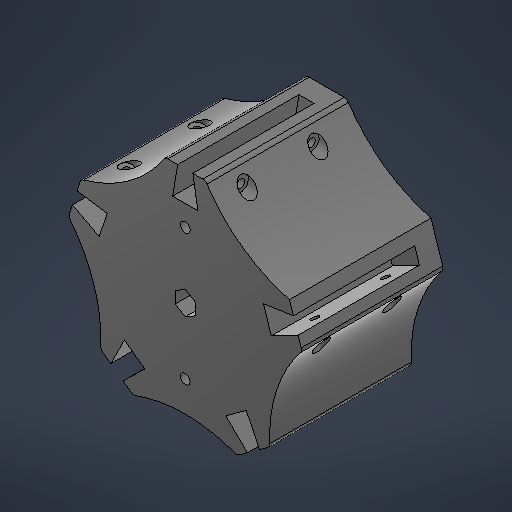
# Autodesk Inventor part: 3DPRINT,HUB
Saved by Autodesk Inventor 2026.1 (Build 301233020, 233B)
## iProperties
Created: 2026-02-05
Part Number: 3DPRINT,HUB
Material: ABS Plastic
Document SubType Name: Modeling
Designer: Owen L
Density: 0.316929 g/cm^3
Appearance: Smooth - Black
Mass: 362.874 g
Surface Area: 937.42 cm^2
Volume: 1144.97 cm^3
Author: Owen L
Autodesk Inventor part; units mm, degrees
ref_plane "XZ Plane" through (0, 0, 0) normal (0, 1, 0) x (-1, 0, 0)
ref_plane "XY Plane" through (0, 0, 0) normal (0, 0, 1) x (1, 0, 0)
sketch "Sketch1" plane through (0, 0, 0) normal (0, 0, 1) x (1, 0, 0)
  line L0 (0, 0) -> (0, 73.025) construction
  line L1 (-12.7, 73.025) -> (12.7, 73.025)
  line L2 (-73.3754, 10.4875) -> (-65.5264, 34.6444)
  line L3 (-32.6485, -66.5433) -> (-53.1975, -51.6136)
  line L4 (53.1975, -51.6136) -> (32.6485, -66.5433)
  line L5 (65.5264, 34.6444) -> (73.3754, 10.4875)
  arc A0 (12.7, 73.025) -> (65.5264, 34.6444) centre (87.7159, 120.7306) ccw
  arc A1 (73.3754, 10.4875) -> (53.1975, -51.6136) centre (141.9273, -46.115) ccw
  arc A2 (32.6485, -66.5433) -> (-32.6485, -66.5433) centre (0, -149.2312) ccw
  arc A3 (-53.1975, -51.6136) -> (-73.3754, 10.4875) centre (-141.9273, -46.115) ccw
  arc A4 (-65.5264, 34.6444) -> (-12.7, 73.025) centre (-87.7159, 120.7306) ccw
  point P0 (65.5264, 34.6444)
  dimension "d0" = 73.025
  dimension "d1" = 25.4
  dimension "d4" = 360
  dimension "d6" = 88.9
  constraints: 12 end point, 10 point on circle, 5 centre point, 4 equal radius, 1 coincident, 1 horizontal, 1 midpoint, 1 vertical, 16 other
  measures "d0" distance of L0.start L0.end
  measures "d1" distance of L1.start L1.end
  measures "d6" radius of A0
extrude "Extrusion5" add sketch "Sketch1" along normal mid plane 88.9
ref_plane "Work Plane5" through (0, 0, 44.45) normal (0, 0, 1) x (1, 0, 0)
sketch "Sketch7" plane through (0, 0, 44.45) normal (0, 0, 1) x (1, 0, 0)
  line L0 (12.7, 73.025) -> (-12.7, 73.025) projected
  line L1 (0, 0) -> (0, 73.025) construction
  line L2 (-4.7625, 73.025) -> (-7.9375, 54.2414)
  line L3 (-7.9375, 54.2414) -> (7.9375, 54.2414)
  line L4 (7.9375, 54.2414) -> (4.7625, 73.025)
  dimension "d121" = 19.05
  dimension "d122" = 15.875
  dimension "d147" = 9.525
  constraints: 8 end point, 2 point on line, 1 equal length, 1 midpoint, 1 other
  measures "d121" distance of L2.start L2.end
  measures "d122" distance of L2.end L3.end
  measures "d147" distance of L2.start L4.end
extrude "Extrusion6" cut sketch "Sketch7" against normal blind 76.2
pattern_circular "Circular Pattern3" count 5 over 360 about axis through (0, 0, -10) along (0, 0, 1) of "Extrusion6"
fillet "Fillet3" radius 3.175 9 edges at (-73.3754, 10.4875, 0) (-65.5264, 34.6444, 0) (-12.7, 73.025, 0) (-53.1975, -51.6136, 0) (-32.6485, -66.5433, 0) (32.6485, -66.5433, 0) (53.1975, -51.6136, 0) (73.3754, 10.4875, 0) (12.7, 73.025, 0)
sketch "Sketch9" plane through (0, 0, -44.45) normal (0, 0, -1) x (-1, 0, 0)
  point P0 (0, 0)
  point P1 (0, -44.45)
  point P2 (38.4948, -22.225)
  point P3 (38.4948, 22.225)
  point P4 (0, 44.45)
  point P5 (-38.4948, 22.225)
  point P6 (-38.4948, -22.225)
  dimension "d93" = 44.45
  dimension "d96" = 360
  constraints: 1 vertical alignment, 7 other
  measures "d93" distance of point (0, 0) point (0, -44.45)
hole "Hole1" at (0, -44.45, -44.45) at (-38.4948, -22.225, -44.45) at (-38.4948, 22.225, -44.45) at (0, 44.45, -44.45) at (38.4948, 22.225, -44.45) at (38.4948, -22.225, -44.45) direction (0, 0, 1) diameter 6.12 depth 12.7 tip angle 118
sketch "Sketch10" plane through (0, 0, 44.45) normal (0, 0, 1) x (1, 0, 0)
  line L0 (0, 41.275) -> (0, 0) construction
  point P0 (0, -41.275)
  dimension "d107" = 360
  dimension "d109" = 41.275
  constraints: 2 end point, 1 vertical, 3 other
  measures "d109" distance of L0.start L0.end
hole "Hole2" at (0, 41.275, 44.45) at (0, -41.275, 44.45) direction (0, 0, -1) diameter 6.12 depth 12.7 tip angle 118
sketch "Sketch11" plane through (0, 0, -44.45) normal (0, 0, -1) x (-1, 0, 0)
  line L0 (-6.4135, -3.7028) -> (-6.4135, 3.7028)
  line L1 (-6.4135, 3.7028) -> (0, 7.4057)
  line L2 (0, 7.4057) -> (6.4135, 3.7028)
  line L3 (6.4135, 3.7028) -> (6.4135, -3.7028)
  line L4 (6.4135, -3.7028) -> (0, -7.4057)
  line L5 (0, -7.4057) -> (-6.4135, -3.7028)
  point P0 (0, 0)
  point P1 (0, 0)
  dimension "d118" = 12.827
  constraints: 12 end point, 1 coincident, 1 vertical, 13 other
  measures "d118" distance between parallel lines of L3 L0
extrude "Extrusion8" cut sketch "Sketch11" against normal through all
ref_plane "Work Plane6" through (38.1, 0, 0) normal (1, 0, 0) x (0, 1, 0)
sketch "Sketch12" plane through (38.1, 0, 0) normal (1, 0, 0) x (0, 1, 0)
  line L0 (71.6045, -44.45) -> (35.0827, -44.45) projected
  circle A0 centre (63.5, 25.4) radius 2.5527
  circle A1 centre (63.5, -19.05) radius 2.5527
  point P0 (0, 0)
  dimension "d123" = 63.5
  dimension "d124" = 25.4
  dimension "d125" = 44.45
  dimension "d127" = 5.1054
  constraints: 2 centre point, 2 coincident, 1 equal radius, 1 vertical alignment
  measures "d123" horizontal distance of point (0, 0) point (63.5, -19.05)
  measures "d124" distance from line of L0 point (63.5, -19.05)
  measures "d125" distance of point (63.5, -19.05) point (63.5, 25.4)
  measures "d127" diameter of A0
hole "Hole3" at (38.1, 63.5, 25.4) at (38.1, 63.5, -19.05) direction (-1, 0, 0) diameter 4.9784 depth 34.925 tip angle 118 counterbore diameter 9.779 counterbore depth 22.352
ref_plane "Work Plane7" through (-38.1, 0, 0) normal (1, 0, 0) x (0, 1, 0)
sketch "Sketch13" plane through (-38.1, 0, 0) normal (1, 0, 0) x (0, 1, 0)
  circle A0 centre (63.5, -19.05) radius 2.4892 projected
  circle A1 centre (63.5, 25.4) radius 2.4892 projected
  point P0 (0, 0)
  point P1 (61.0108, 25.4)
  point P2 (61.0108, 25.4)
  point P3 (76.2, -16.5608)
  point P4 (76.2, -21.5392)
  point P5 (76.2, 27.8892)
  point P6 (76.2, 22.9108)
  constraints: 2 coincident, 2 other
hole "Hole4" [suppressed]
pattern_circular "Circular Pattern4" count 5 over 360 about axis through (0, 0, -10) along (0, 0, 1) of "Hole3"
body "Solid3"
